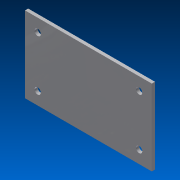
# Autodesk Inventor part: Support_Front
Saved by Autodesk Inventor 2013 (Build 170138000, 138)
## iProperties
Created: 2013-07-13
Part Number: Support_Front
Material: Aluminum 6061
Document SubType Name: Modeling
Designer: orange
Density: 1 g/cm^3
Author: orange
Autodesk Inventor part; units mm, degrees
ref_plane "YZ Plane" through (0, 0, 0) normal (1, 0, 0) x (0, 1, 0)
ref_plane "XZ Plane" through (0, 0, 0) normal (0, 1, 0) x (-1, 0, 0)
ref_plane "XY Plane" through (0, 0, 0) normal (0, 0, 1) x (1, 0, 0)
sketch "Sketch1" plane through (0, 0, 0) normal (0, 0, 1) x (1, 0, 0)
  line L0 (0, 0) -> (127, 0)
  line L1 (127, 0) -> (127, 76.2)
  line L2 (127, 76.2) -> (0, 76.2)
  line L3 (0, 76.2) -> (0, 0)
  dimension "d0" = 127
  dimension "d2" = 76.2
  constraints: 8 end point, 2 parallel, 1 horizontal, 1 perpendicular
  measures "d0" distance of L1.end L2.end
  measures "d2" distance of L2.end L0.start
extrude "Extrusion1" add sketch "Sketch1" along normal blind 3.175
sketch "Sketch2" plane through (0, 0, 3.175) normal (0, 0, 1) x (1, 0, 0)
  line L0 (0, 0) -> (127, 0) projected
  line L1 (127, 0) -> (127, 76.2) projected
  point P0 (114.3, 12.7)
  dimension "d5" = 12.7
  dimension "d6" = 12.7
  measures "d5" distance from line of point (114.3, 12.7) L1
  measures "d6" distance from line of L0 point (114.3, 12.7)
hole "Hole1" at (114.3, 12.7, 3.175) direction (0, 0, -1) diameter 6.35 end through all
sketch "Sketch3" plane through (0, 0, 3.175) normal (0, 0, 1) x (1, 0, 0)
  circle A0 centre (114.3, 12.7) radius 3.175 projected
  line L0 (127, 76.2) -> (0, 76.2) projected
  point P0 (114.3, 63.5)
  dimension "d14" = 12.7
  dimension "d15" = 50.8
  measures "d14" distance from line of point (114.3, 63.5) L0
  measures "d15" distance of A0.centre point (114.3, 63.5)
hole "Hole2" at (114.3, 63.5, 3.175) direction (0, 0, -1) diameter 6.35 end through all
sketch "Sketch4" plane through (0, 0, 3.175) normal (0, 0, 1) x (1, 0, 0)
  line L0 (0, 0) -> (127, 0) projected
  line L1 (127, 76.2) -> (0, 76.2) projected
  line L2 (0, 76.2) -> (0, 0) projected
  point P0 (12.7, 63.5)
  point P1 (12.7, 12.7)
  dimension "d23" = 12.7
  dimension "d24" = 12.7
  dimension "d25" = 12.7
  dimension "d26" = 12.7
  measures "d23" distance from line of L2 point (12.7, 12.7)
  measures "d24" distance from line of L0 point (12.7, 12.7)
  measures "d25" distance from line of point (12.7, 63.5) L1
  measures "d26" distance from line of L2 point (12.7, 63.5)
hole "Hole3" at (12.7, 63.5, 3.175) at (12.7, 12.7, 3.175) direction (0, 0, -1) diameter 6.35 end through all
body "Solid1"
